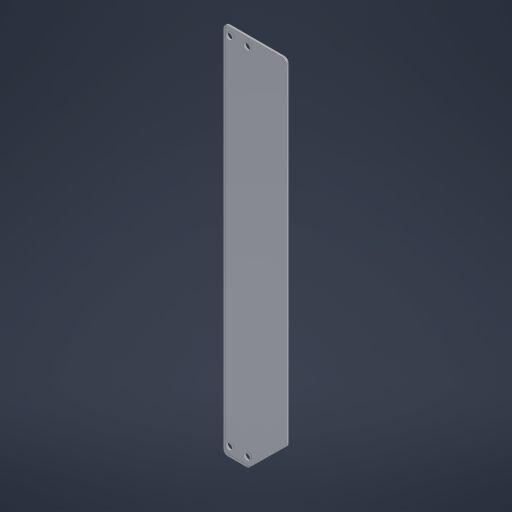
# Autodesk Inventor part: wingplexi
Saved by Autodesk Inventor 2023 (Build 270158000, 158)
## iProperties
Created: 2023-08-07
Part Number: wingplexi
Material: Generic
Document SubType Name: Modeling
Designer: srbel
Density: 1 g/cm^3
Appearance: Clear - White
Author: srbel
Autodesk Inventor part; units mm, degrees
ref_plane "YZ Plane" through (0, 0, 0) normal (1, 0, 0) x (0, 1, 0)
ref_plane "XZ Plane" through (0, 0, 0) normal (0, 1, 0) x (-1, 0, 0)
ref_plane "XY Plane" through (0, 0, 0) normal (0, 0, 1) x (1, 0, 0)
sketch "Sketch1" plane through (0, 0, 0) normal (0, 0, 1) x (1, 0, 0)
  circle A0 centre (3.9687, -260.35) radius 2.1844
  circle A1 centre (16.6687, -260.35) radius 2.1844
  circle A2 centre (3.9687, -6.35) radius 2.1844
  circle A3 centre (16.6687, -6.35) radius 2.1844
  line L0 (3.175, -266.7) -> (8.0073, -266.7)
  line L1 (12.6301, -266.7) -> (16.4968, -266.7)
  line L2 (41.8702, 0) -> (3.175, 0)
  line L3 (3.175, -266.7) -> (16.4968, -266.7)
  line L4 (45.0452, -238.4496) -> (45.0452, -3.175)
  line L5 (41.8702, 0) -> (3.175, 0)
  line L6 (0, -3.175) -> (0, -263.525)
  circle A4 centre (3.9687, -260.35) radius 2.1844
  circle A5 centre (16.6687, -260.35) radius 2.1844
  circle A6 centre (3.9687, -6.35) radius 2.1844
  circle A7 centre (16.6687, -6.35) radius 2.1844
  arc A8 (0, -263.525) -> (3.175, -266.7) centre (3.175, -263.525) ccw
  arc A9 (3.175, 0) -> (0, -3.175) centre (3.175, -3.175) ccw
  arc A10 (45.0452, -3.175) -> (41.8702, 0) centre (41.8702, -3.175) ccw
  line L7 (18.7286, -265.7833) -> (44.1019, -240.7079)
  arc A11 (16.4968, -266.7) -> (18.7286, -265.7833) centre (16.4968, -263.525) ccw
  arc A12 (44.1019, -240.7079) -> (45.0452, -238.4496) centre (41.8702, -238.4496) ccw
  point P0 (0, 0)
  point P1 (18.3752, -266.7)
  point P2 (19.0379, -265.4777)
  point P3 (21.2768, -266.7)
  point P4 (45.0452, -243.1716)
  point P5 (43.8497, -240.9572)
  dimension "d5" = 3.175
  constraints: 16 end point, 13 centre point, 10 point on circle, 10 tangent, 7 equal radius, 4 coincident, 4 point on line, 1 perpendicular
  measures "d5" radius of A11
extrude "Extrusion1" add sketch "Sketch1" along normal blind 1.5875
body "Solid1"
